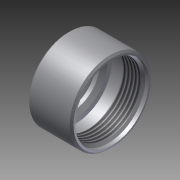
# Autodesk Inventor part: 13_0204_032
Saved by Autodesk Inventor 2012 SP1 (Build 160190100, 190)
## iProperties
Created: 2013-04-04
Part Number: 13_0204_032
Material: Default
Document SubType Name: Modeling
Designer: vogel
Density: 1 g/cm^3
Author: vogel
Autodesk Inventor part; units mm, degrees
ref_plane "YZ Plane" through (0, 0, 0) normal (1, 0, 0) x (0, 1, 0)
ref_plane "XZ Plane" through (0, 0, 0) normal (0, 1, 0) x (-1, 0, 0)
ref_plane "XY Plane" through (0, 0, 0) normal (0, 0, 1) x (1, 0, 0)
sketch "Skizze1" plane through (0, 0, 0) normal (0, 0, 1) x (1, 0, 0)
  line L0 (-14.4, 0) -> (2.4, 0) projected
  line L1 (0, -2.2) -> (0, 13.2) projected
  line L2 (0, 10) -> (-1, 10)
  line L3 (-1, 10) -> (-2, 9)
  line L4 (-2, 9) -> (-6, 9)
  line L5 (-6, 9) -> (-7, 10)
  line L6 (-7, 10) -> (-10, 10)
  line L7 (-10, 10) -> (-10, 8.75)
  line L8 (-0.5, 11) -> (-11.5, 11)
  line L9 (-12, 10.5) -> (-12, 7.75)
  line L10 (-12, 7.75) -> (-11, 7.75)
  line L11 (-11, 7.75) -> (-10, 8.75)
  line L12 (-11.5, 11) -> (-12, 10.5)
  line L13 (0, 10.5) -> (0, 10)
  line L14 (0, 10.5) -> (-0.5, 11)
  point P0 (0, 0)
  point P1 (0, 11)
  point P2 (-12, 11)
  dimension "d0" = 18
  dimension "d1" = 20
  dimension "d2" = 45
  dimension "d3" = 45
  dimension "d4" = 1
  dimension "d5" = 10
  dimension "d6" = 3
  dimension "d7" = 12
  dimension "d9" = 15.5
  dimension "d10" = 1
  dimension "d11" = 0.5
  dimension "d12" = 0.5
  dimension "d13" = 0.5
  dimension "d14" = 0.5
  dimension "d25" = 17.5
  dimension "d26" = 1
  constraints: 26 end point, 6 perpendicular, 6 point on line, 3 collinear, 2 parallel
  measures "d0" diameter of L4 L0
  measures "d1" diameter of L2 L0
  measures "d2" angle of L3 L2
  measures "d3" angle of L5 L4
  measures "d4" distance of L2.start L2.end
  measures "d5" distance between parallel lines of L7 L1
  measures "d6" distance of L5.end L6.end
  measures "d7" distance of point (0, 11) point (-12, 11)
  measures "d9" diameter of L10 L0
  measures "d10" distance of L9.end L10.end
  measures "d11" distance of L8.end point (-12, 11)
  measures "d12" distance of L9.start point (-12, 11)
  measures "d13" distance of L13.start point (0, 11)
  measures "d14" distance of L8.start point (0, 11)
  measures "d25" diameter of L7.end L0
  measures "d26" distance between parallel lines of L8 L2
revolve "Umdrehung1" add sketch "Skizze1" angle 360 about axis through (-10, 0, 0) along (1, 0, 0)
hole "Bohrung1" at (0, 0, 0) direction (-1, 0, 0) diameter 18.917 depth 8 thread size "M20x1" class "6H" standard "ISO Metric profile"
equation "\"d12\" = d11"
equation "\"d14\" = d13"
